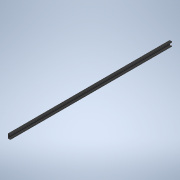
# Autodesk Inventor part: c150x43x15
Saved by Autodesk Inventor 2020 (Build 240168000, 168)
## iProperties
Created: 2022-02-23
Part Number: c150x43x15
Material: Generic
Document SubType Name: Modeling
Designer: super
Density: 1 g/cm^3
Appearance: Default
Author: super
Autodesk Inventor part; units mm, degrees
ref_plane "YZ Plane" through (0, 0, 0) normal (1, 0, 0) x (0, 1, 0)
ref_plane "XZ Plane" through (0, 0, 0) normal (0, 1, 0) x (-1, 0, 0)
ref_plane "XY Plane" through (0, 0, 0) normal (0, 0, 1) x (1, 0, 0)
sketch "Sketch1" plane through (0, 0, 0) normal (0, 0, 1) x (1, 0, 0)
  line L0 (80, 25) -> (80, 0)
  line L1 (80, 0) -> (0, 0)
  line L2 (0, 0) -> (0, 150)
  line L3 (0, 150) -> (80, 150)
  line L4 (80, 150) -> (80, 125)
  line L5 (76.5, 25) -> (76.5, 3.5)
  line L6 (76.5, 3.5) -> (3.5, 3.5)
  line L7 (3.5, 3.5) -> (3.5, 146.5)
  line L8 (3.5, 146.5) -> (76.5, 146.5)
  line L9 (76.5, 146.5) -> (76.5, 125)
  line L10 (76.5, 125) -> (80, 125)
  line L11 (76.5, 25) -> (80, 25)
  dimension "d0" = 80
  dimension "d1" = 150
  dimension "d2" = 25
  dimension "d3" = 25
  dimension "d4" = 3.5
  constraints: 24 end point, 6 perpendicular, 2 point on line, 1 horizontal, 1 parallel, 1 vertical, 4 other
  measures "d0" distance of L0.end L1.end
  measures "d1" distance of L1.end L2.end
  measures "d2" distance of L3.end L4.end
  measures "d3" distance of L0.start L0.end
  measures "d4" distance between parallel lines of L2 L7
extrude "Extrusion1" add sketch "Sketch1" against normal blind 5740
body "Solid1"
